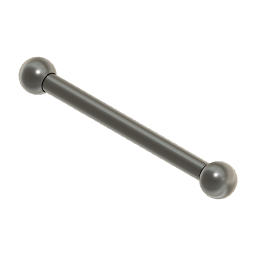
Part III - Spindle v1 (Autodesk Fusion 360 design; units mm, degrees)
Autodesk Fusion 360 part; units mm, degrees
note: some values were not read from the file. Set by a fixed rule: which sketch regions a step uses.
sketch "Sketch1" plane through (0, 0, 0) normal (0, 1, 0) x (1, 0, 0)
  line L0 (0, 0) -> (87.31, 0)
  line L1 (87.31, 0) -> (87.31, -4)
  line L2 (87.31, -4) -> (0, -4)
  line L3 (0, -4) -> (0, 0)
  line L4 (0, 0) -> (126.6344, 0)
  arc A0 (86.15, 0) -> (101.15, 0) centre (93.65, 0) ccw
  arc A1 (-13.84, 0) -> (1.16, 0) centre (-6.34, 0) ccw
  line L5 (0, 0) -> (-20.0914, 0)
  dimension "d1" = 87.31
  dimension "d3" = 15
  dimension "d4" = 6.34
  dimension "d6" = 15
  dimension "d7" = 6.34
  constraint horizontal L0
  constraint vertical L1
  constraint horizontal L2
  constraint vertical L3
  constraint coincident L0.start L3.end
  constraint horizontal L4
  constraint coincident L4 A0.end
  constraint coincident L0 A0.start
  constraint coincident L0 A1.end
  constraint coincident L4 A1.start
  constraint coincident A1.centre L4
  constraint vertical L0.start L3.end
  constraint horizontal L0.start A1.centre
  constraint coincident A0.centre L4
  constraint perpendicular L3 L5
  measures "d1" distance of L0.start L0.end
  measures "d3" diameter of A1
  measures "d4" distance of L3 A1.centre
  measures "d6" diameter of A0
  measures "d7" distance of L1 A0.centre
revolve "Revolve1" add sketch "Sketch1" angle 360 about axis through (0, 0, 0) along (1, 0, 0)
